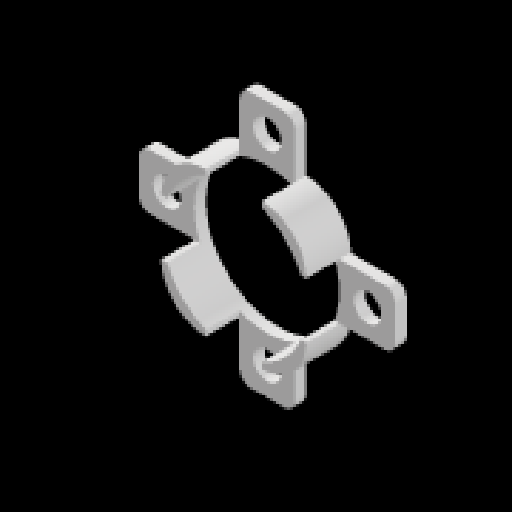
# Autodesk Inventor part: BearingMountMK2
Saved by Autodesk Inventor 2025 (Build 290162000, 162)
## iProperties
Created: 2025-01-19
Part Number: BearingMountMK2
Material: Generic
Document SubType Name: Modeling
Designer: Trevor
Density: 1 g/cm^3
Appearance: Default
Author: Trevor
Autodesk Inventor part; units mm, degrees
ref_plane "YZ Plane" through (0, 0, 0) normal (1, 0, 0) x (0, 1, 0)
sketch "Sketch1" plane through (0, 0, 0) normal (0, 0, 1) x (1, 0, 0)
  circle A0 centre (95.85, -81.2541) radius 13 projected
  line L0 (108.85, -68.2541) -> (108.85, -94.2541)
  line L1 (82.85, -94.2541) -> (82.85, -68.2541)
  line L2 (82.85, -68.2541) -> (108.85, -68.2541)
  line L3 (82.85, -81.2541) -> (77.85, -81.2541) construction
  line L4 (95.85, -68.2541) -> (95.85, -63.2541) construction
  line L5 (108.85, -81.2541) -> (113.85, -81.2541) construction
  line L6 (108.85, -81.2541) -> (113.85, -81.2541) construction
  line L7 (95.85, -94.2541) -> (95.85, -99.2541) construction
  line L8 (92.85, -58.2541) -> (98.85, -58.2541)
  line L9 (100.85, -60.2541) -> (100.85, -68.2541)
  line L10 (100.85, -68.2541) -> (90.85, -68.2541)
  line L11 (90.85, -68.2541) -> (90.85, -60.2541)
  line L12 (90.85, -58.2541) -> (100.85, -68.2541) construction
  line L13 (100.85, -58.2541) -> (90.85, -68.2541) construction
  line L14 (116.85, -76.2541) -> (108.85, -76.2541)
  line L15 (108.85, -76.2541) -> (108.85, -86.2541)
  line L16 (108.85, -86.2541) -> (116.85, -86.2541)
  line L17 (118.85, -84.2541) -> (118.85, -78.2541)
  line L18 (118.85, -76.2541) -> (108.85, -86.2541) construction
  line L19 (108.85, -76.2541) -> (118.85, -86.2541) construction
  line L20 (92.85, -104.2541) -> (98.85, -104.2541)
  line L21 (100.85, -102.2541) -> (100.85, -94.2541)
  line L22 (95.85, -94.2541) -> (90.85, -94.2541)
  line L23 (90.85, -94.2541) -> (90.85, -102.2541)
  line L24 (90.85, -104.2541) -> (100.85, -94.2541) construction
  line L25 (100.85, -104.2541) -> (90.85, -94.2541) construction
  line L26 (74.85, -86.2541) -> (82.85, -86.2541)
  line L27 (82.85, -86.2541) -> (82.85, -76.2541)
  line L28 (82.85, -76.2541) -> (74.85, -76.2541)
  line L29 (72.85, -78.2541) -> (72.85, -84.2541)
  line L30 (72.85, -86.2541) -> (82.85, -76.2541) construction
  line L31 (82.85, -86.2541) -> (72.85, -76.2541) construction
  circle A1 centre (77.85, -81.2541) radius 2.5
  circle A2 centre (95.85, -63.2541) radius 2.5
  circle A3 centre (113.85, -81.2541) radius 2.5
  circle A4 centre (95.85, -99.2541) radius 2.5
  line L32 (108.85, -94.2541) -> (95.85, -94.2541)
  line L33 (90.85, -94.2541) -> (82.85, -94.2541)
  arc A5 (92.85, -58.2541) -> (90.85, -60.2541) centre (92.85, -60.2541) ccw
  arc A6 (100.85, -60.2541) -> (98.85, -58.2541) centre (98.85, -60.2541) ccw
  arc A7 (118.85, -78.2541) -> (116.85, -76.2541) centre (116.85, -78.2541) ccw
  arc A8 (116.85, -86.2541) -> (118.85, -84.2541) centre (116.85, -84.2541) ccw
  arc A9 (98.85, -104.2541) -> (100.85, -102.2541) centre (98.85, -102.2541) ccw
  arc A10 (90.85, -102.2541) -> (92.85, -104.2541) centre (92.85, -102.2541) ccw
  arc A11 (72.85, -84.2541) -> (74.85, -86.2541) centre (74.85, -84.2541) ccw
  arc A12 (74.85, -76.2541) -> (72.85, -78.2541) centre (74.85, -78.2541) ccw
  point P0 (0, 0)
  dimension "d0" = 5
  dimension "d1" = 5
  dimension "d2" = 5
  dimension "d3" = 0
  dimension "d4" = 5
  dimension "d5" = 10
  dimension "d6" = 5
  dimension "d7" = 5
  dimension "d8" = 5
  dimension "d9" = 5
  dimension "d10" = 2
  constraints: 68 end point, 21 point on line, 16 point on circle, 16 tangent, 12 centre point, 11 midpoint, 8 parallel, 7 equal radius, 7 horizontal, 5 coincident, 4 perpendicular, 2 vertical, 1 collinear, 9 other
  measures "d0" distance of L3.start L3.end
  measures "d1" distance of L4.start L4.end
  measures "d2" distance of L5.start L5.end
  measures "d3" distance between parallel lines of L5 L6
  measures "d4" distance of L7.start L7.end
  measures "d5" distance of L9.end L10.end
  measures "d6" diameter of A1
  measures "d7" diameter of A2
  measures "d8" diameter of A3
  measures "d9" diameter of A4
  measures "d10" radius of A5
ref_plane "Work Plane1" through (82.85, -94.2541, 8) normal (0, 0, 1) x (1, 0, 0)
extrude "Extrusion1" add sketch "Sketch1" along normal blind 2 contours L22 L33 L1 A0 | L32 L21 A9 L20 A10 L23 L22 | A0 L0 L32 | A0 L2 L0 | L0 L14 A7 L17 A8 L16 | L1 L2 A0 | L1 L26 A11 L29 A12 L28 | L2 L11 A5 L8 A6 L9
fillet "Fillet1" radius 8 4 edges at (108.85, -68.2541, 1) (82.85, -68.2541, 1) (82.85, -94.2541, 1) (108.85, -94.2541, 1)
sketch "Sketch2" plane through (0, 0, 2) normal (0, 0, 1) x (1, 0, 0)
  arc A0 (100.85, -94.2541) -> (108.85, -86.2541) centre (100.85, -86.2541) ccw projected
  line L0 (108.85, -86.2541) -> (116.85, -86.2541) projected
  arc A1 (116.85, -86.2541) -> (118.85, -84.2541) centre (116.85, -84.2541) ccw projected
  line L1 (118.85, -84.2541) -> (118.85, -78.2541) projected
  arc A2 (118.85, -78.2541) -> (116.85, -76.2541) centre (116.85, -78.2541) ccw projected
  line L2 (116.85, -76.2541) -> (108.85, -76.2541) projected
  arc A3 (108.85, -76.2541) -> (100.85, -68.2541) centre (100.85, -76.2541) ccw projected
  line L3 (100.85, -68.2541) -> (100.85, -60.2541) projected
  arc A4 (100.85, -60.2541) -> (98.85, -58.2541) centre (98.85, -60.2541) ccw projected
  line L4 (98.85, -58.2541) -> (92.85, -58.2541) projected
  arc A5 (92.85, -58.2541) -> (90.85, -60.2541) centre (92.85, -60.2541) ccw projected
  line L5 (90.85, -60.2541) -> (90.85, -68.2541) projected
  arc A6 (90.85, -68.2541) -> (82.85, -76.2541) centre (90.85, -76.2541) ccw projected
  line L6 (82.85, -76.2541) -> (74.85, -76.2541) projected
  arc A7 (74.85, -76.2541) -> (72.85, -78.2541) centre (74.85, -78.2541) ccw projected
  line L7 (72.85, -78.2541) -> (72.85, -84.2541) projected
  arc A8 (72.85, -84.2541) -> (74.85, -86.2541) centre (74.85, -84.2541) ccw projected
  line L8 (74.85, -86.2541) -> (82.85, -86.2541) projected
  arc A9 (82.85, -86.2541) -> (90.85, -94.2541) centre (90.85, -86.2541) ccw projected
  line L9 (90.85, -94.2541) -> (90.85, -102.2541) projected
  arc A10 (90.85, -102.2541) -> (92.85, -104.2541) centre (92.85, -102.2541) ccw projected
  line L10 (92.85, -104.2541) -> (98.85, -104.2541) projected
  arc A11 (98.85, -104.2541) -> (100.85, -102.2541) centre (98.85, -102.2541) ccw projected
  line L11 (100.85, -102.2541) -> (100.85, -94.2541) projected
  circle A12 centre (95.85, -99.2541) radius 2.5 projected
  circle A13 centre (113.85, -81.2541) radius 2.5 projected
  circle A14 centre (95.85, -63.2541) radius 2.5 projected
  circle A15 centre (77.85, -81.2541) radius 2.5 projected
  circle A16 centre (95.85, -81.2541) radius 13 projected
  line L12 (90.85, -68.2541) -> (90.85, -69.2541)
  line L13 (100.85, -68.2541) -> (100.85, -69.2541)
  line L14 (108.85, -76.2541) -> (107.85, -76.2541)
  line L15 (108.85, -86.2541) -> (107.85, -86.2541)
  line L16 (100.85, -94.2541) -> (100.85, -93.2541)
  line L17 (90.85, -94.2541) -> (90.85, -93.2541)
  line L18 (82.85, -86.2541) -> (83.85, -86.2541)
  line L19 (82.85, -76.2541) -> (83.85, -76.2541)
  circle A17 centre (95.85, -81.2541) radius 13 projected
  point P0 (0, 0)
  constraints: 16 end point, 4 point on line, 2 vertical, 1 parallel, 1 perpendicular, 10 other
ref_plane "Work Plane2" through (82.85, -94.2541, 8) normal (0, 0, 1) x (1, 0, 0)
extrude "Extrusion2" add sketch "Sketch2" along normal up to surface (6 mm away) contours L16 A16 L15 A0 | L17 A9 L18 A16 | A16 L13 A3 L14 | L19 A6 L12 A16
body "Solid1"
